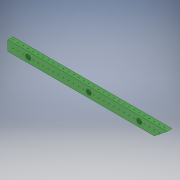
# Autodesk Inventor part: Kermit Frame1
Saved by Autodesk Inventor 2018.2 (Build 222227000, 227)
## iProperties
Created: 2018-02-01
Part Number: Kermit Frame1
Material: Aluminum 6061
Document SubType Name: Modeling
Designer: lopez.xavier
Density: 2.7 g/cm^3
Appearance: Smooth - Dark Forest Green
Author: lopez.xavier
Autodesk Inventor part; units mm, degrees
ref_plane "YZ Plane" through (0, 0, 0) normal (1, 0, 0) x (0, 1, 0)
ref_plane "XZ Plane" through (0, 0, 0) normal (0, 1, 0) x (-1, 0, 0)
ref_plane "XY Plane" through (0, 0, 0) normal (0, 0, 1) x (1, 0, 0)
sketch "Sketch1" plane through (0, 0, 0) normal (0, 0, 1) x (1, 0, 0)
  line L0 (0, 0) -> (800.1, 0)
  line L1 (800.1, 0) -> (800.1, 50.8)
  line L2 (800.1, 50.8) -> (0, 50.8)
  line L3 (0, 50.8) -> (0, 0)
  dimension "d0" = 800.1
  dimension "d1" = 50.8
  constraints: 8 end point, 2 parallel, 1 horizontal, 1 perpendicular
  measures "d0" distance of L1.end L2.end
  measures "d1" distance of L0.end L1.end
extrude "Extrusion1" add sketch "Sketch1" along normal blind 25.4
sketch "Sketch2" plane through (0, 0, 25.4) normal (0, 0, 1) x (1, 0, 0)
  line L0 (0, 0) -> (800.1, 0) projected
  line L1 (800.1, 0) -> (800.1, 50.8) projected
  line L2 (736.6, 0) -> (800.1, 50.8)
  line L3 (736.6, 0) -> (800.1, 0)
  line L4 (800.1, 0) -> (800.1, 50.8)
  dimension "d4" = 63.5
  constraints: 6 end point, 1 horizontal, 1 perpendicular, 1 point on line
  measures "d4" distance of L0.end L2.start
extrude "Extrusion2" cut sketch "Sketch2" against normal blind 25.4
sketch "Sketch3" plane through (0, 0, 0) normal (-1, 0, 0) x (0, 0, 1)
  line L0 (3.175, 47.625) -> (22.225, 47.625)
  line L1 (22.225, 47.625) -> (22.225, 3.175)
  line L2 (22.225, 3.175) -> (3.175, 3.175)
  line L3 (3.175, 3.175) -> (3.175, 47.625)
  line L4 (25.4, 50.8) -> (25.4, 0) projected
  line L5 (0, 50.8) -> (25.4, 50.8) projected
  line L6 (0, 0) -> (25.4, 0) projected
  line L7 (0, 50.8) -> (0, 0) projected
  dimension "d7" = 3.175
  dimension "d8" = 3.175
  dimension "d9" = 3.175
  dimension "d10" = 3.175
  constraints: 8 end point, 2 parallel, 1 horizontal, 1 perpendicular
  measures "d7" distance between parallel lines of L4 L1
  measures "d8" distance between parallel lines of L5 L0
  measures "d9" distance between parallel lines of L6 L2
  measures "d10" distance between parallel lines of L7 L3
extrude "Extrusion3" cut sketch "Sketch3" against normal blind 2540 contours L0 L1 L2 L3
sketch "Sketch4" plane through (0, 0, 25.4) normal (0, 0, 1) x (1, 0, 0)
  circle A0 centre (25.4, 25.4) radius 1.9685
  line L0 (800.1, 50.8) -> (0, 50.8) projected
  line L1 (0, 50.8) -> (0, 0) projected
  circle A1 centre (50.8, 25.4) radius 1.9685
  circle A2 centre (76.2, 25.4) radius 1.9685
  circle A3 centre (101.6, 25.4) radius 1.9685
  circle A4 centre (127, 25.4) radius 1.9685
  circle A5 centre (152.4, 25.4) radius 1.9685
  circle A6 centre (177.8, 25.4) radius 1.9685
  circle A7 centre (203.2, 25.4) radius 1.9685
  circle A8 centre (228.6, 25.4) radius 1.9685
  circle A9 centre (254, 25.4) radius 1.9685
  circle A10 centre (279.4, 25.4) radius 1.9685
  circle A11 centre (304.8, 25.4) radius 1.9685
  circle A12 centre (330.2, 25.4) radius 1.9685
  circle A13 centre (355.6, 25.4) radius 1.9685
  circle A14 centre (381, 25.4) radius 1.9685
  circle A15 centre (406.4, 25.4) radius 1.9685
  circle A16 centre (431.8, 25.4) radius 1.9685
  circle A17 centre (457.2, 25.4) radius 1.9685
  circle A18 centre (482.6, 25.4) radius 1.9685
  circle A19 centre (508, 25.4) radius 1.9685
  circle A20 centre (533.4, 25.4) radius 1.9685
  circle A21 centre (558.8, 25.4) radius 1.9685
  circle A22 centre (584.2, 25.4) radius 1.9685
  circle A23 centre (609.6, 25.4) radius 1.9685
  circle A24 centre (635, 25.4) radius 1.9685
  circle A25 centre (660.4, 25.4) radius 1.9685
  circle A26 centre (685.8, 25.4) radius 1.9685
  circle A27 centre (711.2, 25.4) radius 1.9685
  circle A28 centre (736.6, 25.4) radius 1.9685
  circle A29 centre (762, 25.4) radius 1.9685
  dimension "d13" = 3.937
  dimension "d14" = 25.4
  dimension "d15" = 25.4
  dimension "d18" = 25.4
  constraints: 30 centre point, 1 horizontal, 58 other
  measures "d13" diameter of A0
  measures "d14" distance from line of L0 A0.centre
  measures "d15" distance from line of L1 A0.centre
  measures "d18" distance of A0.centre A1.centre
extrude "Extrusion4" cut sketch "Sketch4" against normal blind 254
sketch "Sketch5" plane through (0, 50.8, 25.4) normal (0, 1, 0) x (1, 0, 0)
  circle A0 centre (12.7, 12.7) radius 1.9685
  line L0 (800.1, 0) -> (0, 0) projected
  line L1 (0, 25.4) -> (0, 0) projected
  circle A1 centre (38.1, 12.7) radius 1.9685
  circle A2 centre (63.5, 12.7) radius 1.9685
  circle A3 centre (88.9, 12.7) radius 1.9685
  circle A4 centre (114.3, 12.7) radius 1.9685
  circle A5 centre (139.7, 12.7) radius 1.9685
  circle A6 centre (165.1, 12.7) radius 1.9685
  circle A7 centre (190.5, 12.7) radius 1.9685
  circle A8 centre (215.9, 12.7) radius 1.9685
  circle A9 centre (241.3, 12.7) radius 1.9685
  circle A10 centre (266.7, 12.7) radius 1.9685
  circle A11 centre (292.1, 12.7) radius 1.9685
  circle A12 centre (317.5, 12.7) radius 1.9685
  circle A13 centre (342.9, 12.7) radius 1.9685
  circle A14 centre (368.3, 12.7) radius 1.9685
  circle A15 centre (393.7, 12.7) radius 1.9685
  circle A16 centre (419.1, 12.7) radius 1.9685
  circle A17 centre (444.5, 12.7) radius 1.9685
  circle A18 centre (469.9, 12.7) radius 1.9685
  circle A19 centre (495.3, 12.7) radius 1.9685
  circle A20 centre (520.7, 12.7) radius 1.9685
  circle A21 centre (546.1, 12.7) radius 1.9685
  circle A22 centre (571.5, 12.7) radius 1.9685
  circle A23 centre (596.9, 12.7) radius 1.9685
  circle A24 centre (622.3, 12.7) radius 1.9685
  circle A25 centre (647.7, 12.7) radius 1.9685
  circle A26 centre (673.1, 12.7) radius 1.9685
  circle A27 centre (698.5, 12.7) radius 1.9685
  circle A28 centre (723.9, 12.7) radius 1.9685
  circle A29 centre (749.3, 12.7) radius 1.9685
  circle A30 centre (774.7, 12.7) radius 1.9685
  dimension "d25" = 3.937
  dimension "d26" = 12.7
  dimension "d27" = 12.7
  dimension "d30" = 25.4
  constraints: 31 centre point, 1 horizontal, 60 other
  measures "d25" diameter of A0
  measures "d26" distance from line of L0 A0.centre
  measures "d27" distance from line of L1 A0.centre
  measures "d30" distance of A0.centre A1.centre
extrude "Extrusion5" cut sketch "Sketch5" against normal blind 254
sketch "Sketch6" plane through (0, 0, 25.4) normal (0, 0, 1) x (1, 0, 0)
  circle A0 centre (101.6, 25.4) radius 1.9685 projected
  circle A1 centre (101.6, 25.4) radius 12.7
  circle A2 centre (406.4, 25.4) radius 12.7
  circle A3 centre (660.4, 25.4) radius 12.7
  point P0 (0, 0)
  dimension "d37" = 25.4
  dimension "d38" = 25.4
  dimension "d39" = 25.4
  dimension "d40" = 304.8
  dimension "d41" = 254
  dimension "d42" = 0
  dimension "d43" = 0
  constraints: 3 centre point, 1 coincident
  measures "d37" diameter of A1
  measures "d38" diameter of A2
  measures "d39" diameter of A3
  measures "d40" distance of A1.centre A2.centre
  measures "d41" distance of A3.centre A2.centre
  measures "d42" vertical distance of A1.centre A2.centre
  measures "d43" vertical distance of A2.centre A3.centre
extrude "Extrusion6" cut sketch "Sketch6" against normal blind 25.4
body "Solid1"
